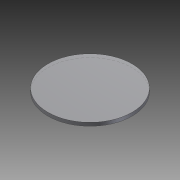
# Autodesk Inventor part: Mirror
Saved by Autodesk Inventor 2012 (Build 160160000, 160)
## iProperties
Created: 2012-11-23
Part Number: Mirror
Material: Default
Document SubType Name: Modeling
Designer: r0oland
Density: 1 g/cm^3
Author: r0oland
Autodesk Inventor part; units mm, degrees
ref_plane "YZ Plane" through (0, 0, 0) normal (1, 0, 0) x (0, 1, 0)
ref_plane "XZ Plane" through (0, 0, 0) normal (0, 1, 0) x (-1, 0, 0)
ref_plane "XY Plane" through (0, 0, 0) normal (0, 0, 1) x (1, 0, 0)
sketch "Sketch1" plane through (0, 0, 0) normal (0, 0, 1) x (1, 0, 0)
  line L0 (0, 9.5652) -> (0, 0)
  line L1 (0, 0) -> (-250, 0)
  arc A0 (-250, 20) -> (0, 9.5652) centre (0, 3009.5652) ccw
  line L2 (-250, 0) -> (-250, 20)
  line L3 (0, 3611.4782) -> (0, -601.913) projected
  line L4 (-300.1306, 0) -> (50.0218, 0) projected
  point P0 (0, 9.5652)
  dimension "d1" = 250
  dimension "d3" = 3000
  dimension "d4" = 20
  constraints: 6 end point, 2 coincident, 2 perpendicular, 2 point on circle, 2 point on line, 1 centre point
  measures "d1" distance of L0.end L1.end
  measures "d3" distance of point (0, 9.565) A0.centre
  measures "d4" distance of L1.end L2.end
revolve "Revolution1" add sketch "Sketch1" angle 360 about axis through (0, 9.5652, 0) along (0, -1, 0)
body "Solid1"
